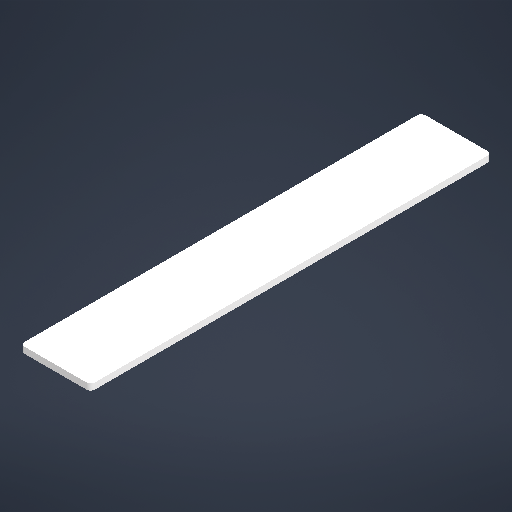
# Autodesk Inventor part: module-lid_switch
Saved by Autodesk Inventor 2025.2 (Build 292293000, 293)
## iProperties
Created: 2025-09-07
Part Number: module-lid_switch
Material: PC/ABS Plastic
Document SubType Name: Modeling
Designer: sam
Density: 1.1 g/cm^3
Appearance: Smooth - White
Author: sam
Autodesk Inventor part; units mm, degrees
ref_plane "YZ Plane" through (0, 0, 0) normal (1, 0, 0) x (0, 1, 0)
ref_plane "XZ Plane" through (0, 0, 0) normal (0, 1, 0) x (-1, 0, 0)
ref_plane "XY Plane" through (0, 0, 0) normal (0, 0, 1) x (1, 0, 0)
sketch "Sketch1" plane through (0, 0, 0) normal (0, 1, 0) x (-1, 0, 0)
  line L0 (-17, -97) -> (17, -97)
  line L1 (17, -97) -> (17, 97)
  line L2 (17, 97) -> (-17, 97)
  line L3 (-17, 97) -> (-17, -97)
  line L4 (-17, -97) -> (17, 97) construction
  line L5 (17, -97) -> (-17, 97) construction
  point P0 (0, 0)
  dimension "d0" = 34
  dimension "d1" = 194
  constraints: 12 end point, 2 midpoint, 2 parallel, 1 horizontal, 1 perpendicular
  measures "d0" distance of L2.end L1.end
  measures "d1" distance between parallel lines of L0 L2
extrude "Extrusion1" add sketch "Sketch1" along normal blind 3
sketch "Sketch2" plane through (0, 0, 0) normal (0, -1, 0) x (1, 0, 0)
  line L0 (14, 94) -> (-14, 94)
  line L1 (-14, 94) -> (-14, -94)
  line L2 (-14, -94) -> (14, -94)
  line L3 (14, -94) -> (14, 94)
  line L4 (14, 94) -> (-14, -94) construction
  line L5 (-14, 94) -> (14, -94) construction
  line L6 (-17, -97) -> (-17, 97) projected
  line L7 (17, -97) -> (-17, -97) projected
  point P0 (0, 0)
  dimension "d4" = 3
  dimension "d5" = 3
  constraints: 12 end point, 2 midpoint, 2 parallel, 1 horizontal, 1 perpendicular
  measures "d4" distance between parallel lines of L6 L1
  measures "d5" distance between parallel lines of L7 L2
extrude "Extrusion2" add sketch "Sketch2" along normal blind 3
fillet "Fillet1" radius 2 8 edges at (17, 1.5, 97) (14, -1.5, 94) (-14, -1.5, 94) (-17, 1.5, 97) (14, -1.5, -94) (17, 1.5, -97) (-17, 1.5, -97) (-14, -1.5, -94)
fillet "Fillet2" radius 0.5 8 edges at (-13.4142, -3, 93.4142) (-14, -3, 0) (-13.4142, -3, -93.4142) (0, -3, -94) (13.4142, -3, -93.4142) (14, -3, 0) (13.4142, -3, 93.4142) (0, -3, 94)
body "Solid1"
